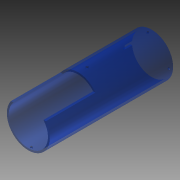
# Autodesk Inventor part: Main_Tubing_Al
Saved by Autodesk Inventor 2011 SP2 (Build 150309200, 309)
## iProperties
Created: 2012-03-18
Part Number: Main_Tubing_Al
Document SubType Name: Modeling
Designer: sungwook
Density: 1 g/cm^3
Author: sungwook
Autodesk Inventor part; units mm, degrees
note: some values were not read from the file. Chosen so that the rebuilt part matches the saved one: direction of "Hole1"; direction of "Hole2".
sketch "Sketch1" plane through (0, 0, 0) normal (0, 0, 1) x (1, 0, 0)
  circle A0 centre (0, 0) radius 14.2875
  circle A1 centre (0, 0) radius 13.0429
  dimension "d0" = 28.575
  dimension "d1" = 26.0858
  constraints: 2 centre point, 2 coincident
  measures "d0" diameter of A0
  measures "d1" diameter of A1
extrude "Extrusion1" add sketch "Sketch1" along normal blind 81.9912
ref_plane "POffset" through (0, 8.3, 0) normal (0, 1, 0) x (-1, 0, 0)
sketch "Sketch2" plane through (0, 8.3, 0) normal (0, 1, 0) x (-1, 0, 0)
  line L0 (11.6294, 81.9912) -> (11.6294, 0) projected
  line L1 (11.6294, 0) -> (10.0612, 0) projected
  line L2 (10.0612, 0) -> (10.0612, 81.9912) projected
  line L3 (10.0612, 81.9912) -> (11.6294, 81.9912) projected
  line L4 (-11.6294, 0) -> (-11.6294, 81.9912) projected
  line L5 (-11.6294, 81.9912) -> (-10.0612, 81.9912) projected
  line L6 (-10.0612, 81.9912) -> (-10.0612, 0) projected
  line L7 (-10.0612, 0) -> (-11.6294, 0) projected
  line L8 (-11.6294, 81.9912) -> (11.6294, 81.9912)
  line L9 (11.6294, 81.9912) -> (11.6294, 48.9912)
  line L10 (11.6294, 48.9912) -> (-11.6294, 48.9912)
  line L11 (-11.6294, 48.9912) -> (-11.6294, 81.9912)
  point P0 (0, 0)
  dimension "d5" = 33
  constraints: 8 end point, 2 parallel, 1 horizontal, 1 perpendicular, 1 point on line
  measures "d5" distance of L9.end L8.end
extrude "Extrusion2" cut sketch "Sketch2" along normal through all contours L0 L10 L2 L3 | L2 L10 L6 L8 | L6 L10 L4 L5
ref_plane "Work Plane2" through (0, 14.2875, 0) normal (0, 1, 0) x (-1, 0, 0)
sketch "Sketch3" plane through (0, 14.2875, 0) normal (0, 1, 0) x (-1, 0, 0)
  line L0 (-14.2875, 0) -> (14.2875, 0) projected
  line L1 (0, -16.3982) -> (0, 98.3894) projected
  point P0 (0, 0)
  point P1 (0, 2.5)
  dimension "d8" = 2.5
  constraints: 1 point on line
  measures "d8" distance from line of L0 point (0, 2.5)
hole "Hole1" at (0, 14.2875, 2.5) direction (0, -1, 0) diameter 1 end up to surface
ref_plane "Work Plane3" through (14.2875, 0, 0) normal (1, 0, 0) x (0, 1, 0)
sketch "Sketch4" plane through (14.2875, 0, 0) normal (1, 0, 0) x (0, 1, 0)
  line L0 (-14.2875, 0) -> (14.2875, 0) projected
  line L1 (0, -16.3982) -> (0, 98.3894) projected
  point P0 (0, 0)
  point P1 (0, 2.5)
  dimension "d16" = 2.5
  constraints: 1 point on line
  measures "d16" distance from line of L0 point (0, 2.5)
hole "Hole2" at (14.2875, 0, 2.5) direction (-1, 0, 0) diameter 1 end up to surface
ref_plane "Work Plane4" through (-14.2875, 0, 0) normal (1, 0, 0) x (0, 1, 0)
sketch "Sketch5" plane through (-14.2875, 0, 0) normal (1, 0, 0) x (0, 1, 0)
  line L0 (-14.2875, 0) -> (14.2875, 0) projected
  line L1 (0, -16.3982) -> (0, 98.3894) projected
  line L2 (1.25, 5) -> (-1.25, 5)
  line L3 (-1.25, 5) -> (-1.25, 0)
  line L4 (-1.25, 0) -> (1.25, 0)
  line L5 (1.25, 0) -> (1.25, 5)
  point P0 (0, 0)
  point P1 (0, 5)
  point P2 (0, 0)
  dimension "d24" = 2.5
  dimension "d25" = 5
  constraints: 8 end point, 2 midpoint, 2 parallel, 1 horizontal, 1 perpendicular, 1 point on line, 1 vertical alignment
  measures "d24" distance of L2.end L2.start
  measures "d25" distance of L4.end L2.start
extrude "Extrusion3" cut sketch "Sketch5" along normal blind 3
ref_plane "Work Plane5" through (0, -14.2875, 0) normal (0, 1, 0) x (-1, 0, 0)
sketch "Sketch6" plane through (0, -14.2875, 0) normal (0, 1, 0) x (-1, 0, 0)
  line L0 (-13.0429, 81.9912) -> (13.0429, 81.9912) projected
  line L1 (0, -16.3982) -> (0, 98.3894) projected
  point P0 (0, 0)
  point P1 (-10.0612, 81.9912)
  point P2 (10.0612, 81.9912)
  point P3 (0, 80.0572)
  dimension "d28" = 1.934
  constraints: 1 point on line
  measures "d28" distance from line of point (0, 80.057) L0
hole "Hole3" at (0, -14.2875, 80.0572) direction (0, 1, 0) diameter 1.1938 end through all
sketch "Sketch7" plane through (0, 14.2875, 0) normal (0, 1, 0) x (-1, 0, 0)
  line L0 (-13.0429, 81.9912) -> (13.0429, 81.9912) projected
  line L1 (0, -16.3982) -> (0, 98.3894) projected
  point P0 (0, 0)
  point P1 (-10.0612, 81.9912)
  point P2 (10.0612, 81.9912)
  point P3 (0, 42.9912)
  dimension "d36" = 39
  constraints: 1 point on line
  measures "d36" distance from line of point (0, 42.991) L0
hole "Hole4" at (0, 14.2875, 42.9912) direction (0, -1, 0) diameter 1.7018 depth 3
equation "\"d5\" = length"
equation "\"POffset\" = 8.3"
equation "\"d4\" = POffset"
equation "\"length\" = 33"
body "Solid1"
